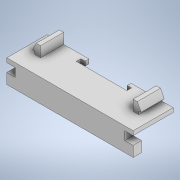
# Autodesk Inventor part: Clip
Saved by Autodesk Inventor 2022.2 (Build 262287000, 287)
## iProperties
Created: 2022-01-22
Part Number: Clip
Material: Generisch
Document SubType Name: Modeling
Designer: hpcwoess
Density: 1 g/cm^3
Appearance: Vorgabe
Author: hpcwoess
Autodesk Inventor part; units mm, degrees
ref_plane "YZ Plane" through (0, 0, 0) normal (1, 0, 0) x (0, 1, 0)
ref_plane "XZ Plane" through (0, 0, 0) normal (0, 1, 0) x (-1, 0, 0)
ref_plane "XY Plane" through (0, 0, 0) normal (0, 0, 1) x (1, 0, 0)
sketch "Skizze1" plane through (0, 0, 0) normal (0, 0, 1) x (1, 0, 0)
  line L0 (-30, 0) -> (30, 0)
  line L1 (30, 0) -> (30, 2)
  line L2 (30, 2) -> (24.75, 2)
  line L3 (24.75, 2) -> (24.75, 3.5)
  line L4 (24.75, 3.5) -> (25.75, 3.5)
  line L5 (25.75, 3.5) -> (24, 7)
  line L6 (24, 7) -> (22, 7)
  line L7 (22, 7) -> (22, 2)
  line L8 (22, 2) -> (-22, 2)
  line L9 (-22, 2) -> (-22, 7)
  line L10 (-22, 7) -> (-24, 7)
  line L11 (-24, 7) -> (-25.75, 3.5)
  line L12 (-25.75, 3.5) -> (-24.75, 3.5)
  line L13 (-24.75, 3.5) -> (-24.75, 2)
  line L14 (-24.75, 2) -> (-30, 2)
  line L15 (-30, 2) -> (-30, 0)
  point P0 (0, 0)
  point P1 (0, 0)
  dimension "d0" = 49.5
  dimension "d1" = 24.75
  dimension "d2" = 5.25
  dimension "d3" = 5.25
  dimension "d4" = 1
  dimension "d5" = 1
  dimension "d6" = 44
  dimension "d7" = 2
  dimension "d8" = 22
  dimension "d9" = 2
  dimension "d10" = 5
  dimension "d11" = 2
  dimension "d12" = 2
  dimension "d13" = 1.5
  constraints: 33 end point, 9 perpendicular, 4 point on line, 2 midpoint, 1 collinear, 1 horizontal, 1 parallel, 1 vertical
  measures "d0" distance of L2.end L13.end
  measures "d1" horizontal distance of point (0, 0) L2.end
  measures "d2" horizontal distance of L2.end L0.end
  measures "d3" horizontal distance of L13.end L0.start
  measures "d4" distance from line of L11.end L13
  measures "d5" distance from line of L4.end L3
  measures "d6" distance between parallel lines of L7 L9
  measures "d7" distance of L9.end L10.end
  measures "d8" distance from line of point (0, 0) L9
  measures "d9" distance from line of L5.end L7
  measures "d10" distance of L6.end L7.end
  measures "d11" distance between parallel lines of L0 L8
  measures "d12" distance between parallel lines of L0 L14
  measures "d13" distance of L12.end L13.end
extrude "Extrusion1" add sketch "Skizze1" along normal blind 11
sketch "Skizze2" plane through (30, 0, 0) normal (1, 0, 0) x (0, 0, -1)
  line L0 (-11, 0) -> (-11, 2) projected
  line L1 (-19, 0) -> (-19, -9)
  line L2 (-19, -9) -> (-15, -9)
  line L3 (-15, -9) -> (-15, -7)
  line L4 (-15, -7) -> (-17, -7)
  line L5 (-17, -7) -> (-17, -5)
  line L6 (-17, -5) -> (-15, -5)
  line L7 (-15, -5) -> (-15, 0)
  line L8 (0, 0) -> (-11, 0) projected
  line L9 (-11, 2) -> (-11, 0) projected
  line L10 (-15, 0) -> (-11, 0)
  line L11 (-11, 2) -> (-11, 7) projected
  line L12 (-11, 0) -> (-11, 2)
  line L13 (-11, 2) -> (-19, 2)
  line L14 (-19, 2) -> (-19, 0)
  point P0 (-11, 1)
  dimension "d16" = 9
  dimension "d17" = 4
  dimension "d18" = 2
  dimension "d19" = 2
  dimension "d20" = 2
  dimension "d23" = 4
  dimension "d24" = 2
  constraints: 22 end point, 6 perpendicular, 2 collinear, 2 point on line, 1 horizontal, 1 midpoint, 1 vertical
  measures "d16" distance of L1.start L1.end
  measures "d17" distance of L1.end L2.end
  measures "d18" distance of L2.end L3.end
  measures "d19" distance of L3.end L4.end
  measures "d20" distance of L4.end L5.end
  measures "d23" distance from line of point (-11, 1) L7
  measures "d24" distance from line of L1.start L13
extrude "Extrusion2" add sketch "Skizze2" against normal up to surface (60 mm away)
sketch "Skizze3" plane through (30, -5, 15) normal (0, 0, -1) x (-1, 0, 0)
  line L0 (60, 7) -> (60, -4) projected
  line L1 (0, 0) -> (60, 0) projected
  line L2 (60, -4) -> (58.5, -4)
  line L3 (58.5, -4) -> (58.5, 0)
  line L4 (58.5, 0) -> (60, 0)
  line L5 (60, 0) -> (60, -4)
  line L6 (0, 7) -> (0, -4) projected
  line L7 (0, -4) -> (1.5, -4)
  line L8 (1.5, -4) -> (1.5, 0)
  line L9 (1.5, 0) -> (0, 0)
  line L10 (0, 0) -> (0, -4)
  line L11 (60, 5) -> (0, 5) projected
  point P0 (30, 5)
  point P1 (30, 5)
  point P2 (1.5, 0)
  dimension "d25" = 57
  dimension "d26" = 28.5
  constraints: 16 end point, 4 parallel, 2 horizontal, 2 perpendicular, 2 point on line, 1 midpoint
  measures "d25" distance between parallel lines of L8 L3
  measures "d26" distance from line of point (30, 5) L8
extrude "Extrusion3" add sketch "Skizze3" against normal up to surface (2 mm away) contours L0 L2 L3 L1 | L1 L8 L7 L6
sketch "Skizze4" plane through (-30, 0, 0) normal (0, -1, 0) x (1, 0, 0)
  line L0 (52, 0) -> (8, 0) projected
  line L1 (20, 0) -> (40, 0)
  line L2 (40, 0) -> (40, 4)
  line L3 (40, 4) -> (20, 4)
  line L4 (20, 4) -> (20, 0)
  line L5 (20, 4) -> (18, 4)
  line L6 (18, 4) -> (18, 1.8)
  line L7 (18, 1.8) -> (20, 1.8)
  line L8 (20, 1.8) -> (20, 4)
  line L9 (40, 4) -> (42, 4)
  line L10 (42, 4) -> (42, 1.8)
  line L11 (42, 1.8) -> (40, 1.8)
  line L12 (40, 1.8) -> (40, 4)
  point P0 (30, 0)
  point P1 (40, 2.9)
  point P2 (41, 1.8)
  point P3 (30, 0)
  dimension "d29" = 20
  dimension "d30" = 2
  dimension "d31" = 2
  dimension "d32" = 2.2
  dimension "d33" = 1.8
  dimension "d34" = 10
  constraints: 24 end point, 6 parallel, 3 horizontal, 3 midpoint, 3 perpendicular, 2 point on line
  measures "d29" distance of L2.end L3.end
  measures "d30" horizontal distance of point (40, 2.9) L9.end
  measures "d31" distance from line of L4 L5.end
  measures "d32" distance of L9.end L10.end
  measures "d33" distance from line of point (41, 1.8) L0
  measures "d34" distance from line of point (30, 0) L4
extrude "Extrusion4" cut sketch "Skizze4" against normal blind 10
sketch "Skizze5" plane through (30, -9, 15) normal (0, 0, -1) x (-1, 0, 0)
  line L0 (0, 11) -> (0, 0) projected
  line L1 (0, 9) -> (60, 9) projected
  line L2 (0, 5) -> (4, 5)
  line L3 (4, 5) -> (4, 9)
  line L4 (4, 9) -> (0, 9)
  line L5 (0, 9) -> (0, 5)
  line L6 (60, 0) -> (60, 9) projected
  line L7 (60, 5) -> (56, 5)
  line L8 (56, 5) -> (56, 9)
  line L9 (56, 9) -> (60, 9)
  line L10 (60, 9) -> (60, 5)
  point P0 (30, 9)
  dimension "d37" = 4
  dimension "d38" = 4
  dimension "d39" = 4
  constraints: 16 end point, 4 parallel, 4 point on line, 2 horizontal, 2 perpendicular, 1 collinear
  measures "d37" distance of L7.start L7.end
  measures "d38" distance between parallel lines of L1 L7
  measures "d39" distance between parallel lines of L0 L3
extrude "Extrusion5" cut sketch "Skizze5" against normal blind 10
equation "\"d1\" = 0.5 * d0"
equation "\"d3\" = d2"
equation "\"d5\" = d4"
equation "\"d8\" = 0.5 * d6"
equation "\"d9\" = d7"
equation "\"d26\" = 0.5 * d25"
equation "\"d31\" = d30"
equation "\"d34\" = 0.5 * d29"
equation "\"d38\" = d37"
equation "\"d39\" = d37"
